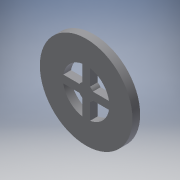
# Autodesk Inventor part: Impeller 1
Saved by Autodesk Inventor 2018 (Build 220112000, 112)
## iProperties
Created: 2018-01-25
Part Number: Impeller 1
Material: Generic
Document SubType Name: Modeling
Designer: Rus
Density: 1 g/cm^3
Appearance: Default
Author: Rus
Autodesk Inventor part; units mm, degrees
ref_plane "YZ Plane" through (0, 0, 0) normal (1, 0, 0) x (0, 1, 0)
ref_plane "XZ Plane" through (0, 0, 0) normal (0, 1, 0) x (-1, 0, 0)
ref_plane "XY Plane" through (0, 0, 0) normal (0, 0, 1) x (1, 0, 0)
sketch "Sketch1" plane through (0, 0, 0) normal (0, 0, 1) x (1, 0, 0)
  circle A0 centre (0, 0) radius 76.2
  dimension "d0" = 152.4
  constraints: 1 centre point, 1 coincident
  measures "d0" diameter of A0
extrude "Extrusion1" add sketch "Sketch1" along normal blind 12.7
sketch "Sketch4" plane through (0, 0, 12.7) normal (0, 0, 1) x (1, 0, 0)
  circle A0 centre (0, 0) radius 38.1
  line L0 (-38.1, 0) -> (38.1, 0) construction
  line L1 (-38.1, -6.35) -> (38.1, -6.35)
  line L2 (38.1, 6.35) -> (-38.1, 6.35)
  arc A1 (-38.1, 6.35) -> (-38.1, -6.35) centre (-38.1, 0) ccw
  arc A2 (38.1, -6.35) -> (38.1, 6.35) centre (38.1, 0) ccw
  line L3 (0, 38.1) -> (0, -38.1) construction
  line L4 (-6.35, 38.1) -> (-6.35, -38.1)
  line L5 (6.35, -38.1) -> (6.35, 38.1)
  arc A3 (6.35, 38.1) -> (-6.35, 38.1) centre (0, 38.1) ccw
  arc A4 (-6.35, -38.1) -> (6.35, -38.1) centre (0, -38.1) ccw
  circle A5 centre (0, 0) radius 12.7
  dimension "d17" = 76.2
  dimension "d18" = 12.7
  dimension "d19" = 12.7
  dimension "d20" = 25.4
  constraints: 16 end point, 10 point on circle, 8 tangent, 6 centre point, 2 coincident, 2 midpoint, 2 parallel, 1 horizontal, 1 perpendicular
  measures "d17" diameter of A0
  measures "d18" diameter of A2
  measures "d19" diameter of A4
  measures "d20" diameter of A5
extrude "Extrusion2" cut sketch "Sketch4" against normal blind 12.7 contours A0 L1 A5 L2 | L2 A5 L5 A0 | A0 L5 A5 L1 | L5 A5 L4 A0 | A0 L4 A5 L5 | L4 A5 L2 A0 | A0 L1 A5 L4 | L2 A5 L1 A0
sketch "Sketch5" plane through (0, 0, 12.7) normal (0, 0, 1) x (1, 0, 0)
  line L0 (-38.1, 0) -> (38.1, 0) construction
  line L1 (-38.1, -6.35) -> (38.1, -6.35)
  line L2 (38.1, 6.35) -> (-38.1, 6.35)
  arc A0 (-38.1, 6.35) -> (-38.1, -6.35) centre (-38.1, 0) ccw
  arc A1 (38.1, -6.35) -> (38.1, 6.35) centre (38.1, 0) ccw
  line L3 (0, -38.1) -> (0, 38.1) construction
  line L4 (6.35, -38.1) -> (6.35, 38.1)
  line L5 (-6.35, 38.1) -> (-6.35, -38.1)
  arc A2 (-6.35, -38.1) -> (6.35, -38.1) centre (0, -38.1) ccw
  arc A3 (6.35, 38.1) -> (-6.35, 38.1) centre (0, 38.1) ccw
  line L6 (0, 0) -> (76.2, 0) construction
  dimension "d23" = 38.1
  dimension "d24" = 12.7
  dimension "d25" = 38.1
  dimension "d26" = 90
  dimension "d27" = 12.7
  constraints: 18 end point, 8 point on circle, 8 tangent, 4 centre point, 2 horizontal, 2 midpoint, 2 parallel, 2 perpendicular
  measures "d23" distance of L6.start L0.end
  measures "d24" diameter of A1
  measures "d25" distance of L6.start L3.end
  measures "d26" angle of L6 L3
  measures "d27" diameter of A3
extrude "Extrusion3" add sketch "Sketch5" against normal blind 12.7
sketch "Sketch6" plane through (0, 0, 12.7) normal (0, 0, 1) x (1, 0, 0)
  line L0 (-82.4889, 47.625) -> (-67.3519, 67.3519) construction
  line L1 (-67.3519, 67.3519) -> (-47.625, 82.4889) construction
  line L2 (-47.625, 82.4889) -> (-24.6525, 92.0044) construction
  line L3 (-24.6525, 92.0044) -> (0, 95.25) construction
  line L4 (0, 95.25) -> (24.6525, 92.0044) construction
  line L5 (24.6525, 92.0044) -> (47.625, 82.4889) construction
  line L6 (47.625, 82.4889) -> (67.3519, 67.3519) construction
  line L7 (67.3519, 67.3519) -> (82.4889, 47.625) construction
  line L8 (82.4889, 47.625) -> (92.0044, 24.6525) construction
  line L9 (92.0044, 24.6525) -> (95.25, 0) construction
  line L10 (95.25, 0) -> (92.0044, -24.6525) construction
  line L11 (92.0044, -24.6525) -> (82.4889, -47.625) construction
  line L12 (82.4889, -47.625) -> (67.3519, -67.3519) construction
  line L13 (67.3519, -67.3519) -> (47.625, -82.4889) construction
  line L14 (47.625, -82.4889) -> (24.6525, -92.0044) construction
  line L15 (24.6525, -92.0044) -> (0, -95.25) construction
  line L16 (0, -95.25) -> (-24.6525, -92.0044) construction
  line L17 (-24.6525, -92.0044) -> (-47.625, -82.4889) construction
  line L18 (-47.625, -82.4889) -> (-67.3519, -67.3519) construction
  line L19 (-67.3519, -67.3519) -> (-82.4889, -47.625) construction
  line L20 (-82.4889, -47.625) -> (-92.0044, -24.6525) construction
  line L21 (-92.0044, -24.6525) -> (-95.25, 0) construction
  line L22 (-95.25, 0) -> (-92.0044, 24.6525) construction
  line L23 (-92.0044, 24.6525) -> (-82.4889, 47.625) construction
  arc A0 (53.8815, 53.8815) -> (19.722, 73.6035) centre (0, 0) ccw
  arc A1 (-6.35, 10.9985) -> (-10.9985, 6.35) centre (0, 0) ccw construction
  line L24 (-10.9985, 6.35) -> (-37.5671, 6.35) construction
  arc A2 (-6.35, 37.5671) -> (-37.5671, 6.35) centre (0, 0) ccw construction
  line L25 (-6.35, 37.5671) -> (-6.35, 10.9985) construction
  arc A3 (-10.9985, -6.35) -> (-6.35, -10.9985) centre (0, 0) ccw construction
  line L26 (-6.35, -10.9985) -> (-6.35, -37.5671) construction
  arc A4 (-37.5671, -6.35) -> (-6.35, -37.5671) centre (0, 0) ccw construction
  line L27 (-37.5671, -6.35) -> (-10.9985, -6.35) construction
  line L28 (6.35, 10.9985) -> (6.35, 37.5671) construction
  arc A5 (37.5671, 6.35) -> (6.35, 37.5671) centre (0, 0) ccw construction
  line L29 (37.5671, 6.35) -> (10.9985, 6.35) construction
  arc A6 (10.9985, 6.35) -> (6.35, 10.9985) centre (0, 0) ccw construction
  circle A7 centre (0, 0) radius 76.2 construction
  line L30 (10.9985, -6.35) -> (37.5671, -6.35) construction
  arc A8 (6.35, -37.5671) -> (37.5671, -6.35) centre (0, 0) ccw construction
  line L31 (6.35, -37.5671) -> (6.35, -10.9985) construction
  arc A9 (6.35, -10.9985) -> (10.9985, -6.35) centre (0, 0) ccw construction
  line L32 (19.722, 73.6035) -> (53.8815, 53.8815) construction
  line L33 (53.8815, 53.8815) -> (73.6035, 19.722) construction
  line L34 (73.6035, 19.722) -> (73.6035, -19.722) construction
  line L35 (73.6035, -19.722) -> (53.8815, -53.8815) construction
  line L36 (53.8815, -53.8815) -> (19.722, -73.6035) construction
  line L37 (19.722, -73.6035) -> (-19.722, -73.6035) construction
  line L38 (-19.722, -73.6035) -> (-53.8815, -53.8815) construction
  line L39 (-53.8815, -53.8815) -> (-73.6035, -19.722) construction
  line L40 (-73.6035, -19.722) -> (-73.6035, 19.722) construction
  line L41 (-73.6035, 19.722) -> (-53.8815, 53.8815) construction
  line L42 (-53.8815, 53.8815) -> (-19.722, 73.6035) construction
  line L43 (-19.722, 73.6035) -> (19.722, 73.6035) construction
  circle A10 centre (0, 0) radius 25.4 construction
  arc A11 (12.7, 21.997) -> (53.8815, 53.8815) centre (16.2647, 59.9299) ccw
  arc A12 (12.7, 21.997) -> (19.722, 73.6035) centre (-11.3465, 51.55) ccw
  line L44 (12.7, 21.997) -> (47.625, 82.4889) construction
  dimension "d35" = 50.8
  dimension "d30" = 190.5
  dimension "d45" = 38.1
  dimension "d46" = 38.1
  constraints: 74 end point, 8 point on circle, 4 coincident, 3 centre point, 1 horizontal, 1 horizontal alignment, 1 perpendicular, 77 other
  measures "d30" distance of L9.end L21.end
  measures "d45" radius of A11
  measures "d46" radius of A12
extrude "Extrusion4" add sketch "Sketch6" along normal blind 12.7
pattern_circular "Circular Pattern1" count 6 over 360 about axis through (0, 0, 0) along (0, 0, 1) of "Extrusion4"
body "Solid1"
